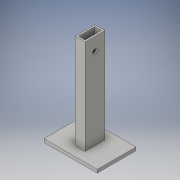
# Autodesk Inventor part: SupportPost
Saved by Autodesk Inventor 2016 SP1 (Build 200210100, 210)
## iProperties
Created: 2016-02-07
Part Number: SupportPost
Material: Generic
Document SubType Name: Modeling
Designer: steele
Density: 1 g/cm^3
Appearance: Default
Author: steele
Autodesk Inventor part; units mm, degrees
ref_plane "YZ Plane" through (0, 0, 0) normal (1, 0, 0) x (0, 1, 0)
ref_plane "XZ Plane" through (0, 0, 0) normal (0, 1, 0) x (-1, 0, 0)
ref_plane "XY Plane" through (0, 0, 0) normal (0, 0, 1) x (1, 0, 0)
sketch "Sketch1" plane through (0, 0, 0) normal (0, 1, 0) x (-1, 0, 0)
  line L0 (50.8, 37.1061) -> (-50.8, 37.1061)
  line L1 (-50.8, 37.1061) -> (-50.8, -37.1061)
  line L2 (-50.8, -37.1061) -> (50.8, -37.1061)
  line L3 (50.8, -37.1061) -> (50.8, 37.1061)
  line L4 (50.8, 37.1061) -> (-50.8, -37.1061) construction
  line L5 (-50.8, 37.1061) -> (50.8, -37.1061) construction
  point P0 (0, 0)
  dimension "d0" = 101.6
  dimension "d1" = 74.2122
  constraints: 12 end point, 2 midpoint, 2 parallel, 1 horizontal, 1 perpendicular
  measures "d0" distance of L0.start L0.end
  measures "d1" distance of L2.end L0.start
extrude "Extrusion1" add sketch "Sketch1" along normal blind 6.35
sketch "Sketch2" plane through (0, 6.35, 0) normal (0, 1, 0) x (1, 0, 0)
  line L0 (-9.525, -19.05) -> (9.525, -19.05)
  line L1 (9.525, -19.05) -> (9.525, 19.05)
  line L2 (9.525, 19.05) -> (-9.525, 19.05)
  line L3 (-9.525, 19.05) -> (-9.525, -19.05)
  line L4 (-9.525, -19.05) -> (9.525, 19.05) construction
  line L5 (9.525, -19.05) -> (-9.525, 19.05) construction
  line L6 (-6.35, -15.875) -> (6.35, -15.875)
  line L7 (6.35, -15.875) -> (6.35, 15.875)
  line L8 (6.35, 15.875) -> (-6.35, 15.875)
  line L9 (-6.35, 15.875) -> (-6.35, -15.875)
  line L10 (-6.35, -15.875) -> (6.35, 15.875) construction
  line L11 (6.35, -15.875) -> (-6.35, 15.875) construction
  point P0 (0, 0)
  dimension "d4" = 19.05
  dimension "d5" = 38.1
  dimension "d6" = 3.175
  dimension "d7" = 3.175
  constraints: 24 end point, 4 midpoint, 4 parallel, 2 horizontal, 2 perpendicular
  measures "d4" distance of L0.start L0.end
  measures "d5" distance of L2.end L0.start
  measures "d6" distance between parallel lines of L0 L6
  measures "d7" distance between parallel lines of L9 L3
extrude "Extrusion2" add sketch "Sketch2" along normal blind 181.5338
sketch "Sketch3" plane through (9.525, 6.35, 19.05) normal (1, 0, 0) x (0, 0, -1)
  circle A0 centre (19.05, 156.1338) radius 4.7625
  line L0 (0, 181.5338) -> (38.1, 181.5338) projected
  point P0 (19.05, -6.35)
  dimension "d10" = 9.525
  dimension "d11" = 25.4
  constraints: 1 centre point
  measures "d10" diameter of A0
  measures "d11" distance from line of A0.centre L0
extrude "Extrusion3" cut sketch "Sketch3" against normal through all
equation "\"d0\" = baseWidth"
equation "\"d2\" = baseThickness"
equation "\"d4\" = postWidth"
equation "\"d5\" = postLength"
equation "\"d6\" = postWallThickness"
equation "\"d7\" = postWallThickness"
equation "\"d8\" = postHeight"
equation "\"d10\" = axelDiam"
equation "\"d11\" = distanceFromTopToAxel"
equation "\"baseWidth\" = 101.6"
equation "\"baseLength\" = 101.6"
equation "\"baseThickness\" = 6.35"
equation "\"postWidth\" = 19.05"
equation "\"postLength\" = 38.1"
equation "\"postWallThickness\" = 3.175"
equation "\"axelDiam\" = 9.525"
equation "\"distanceFromTopToAxel\" = 25.4"
equation "\"heightOfAxelFromAssembly\" = 156.1338"
equation "\"postHeight\" = 181.5338"
body "Solid1"
